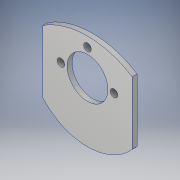
# Autodesk Inventor part: Gear Protection Piece
Saved by Autodesk Inventor 2019.4 (Build 234330000, 330)
## iProperties
Created: 2019-11-02
Part Number: Gear Protection Piece
Material: Aluminum 6061
Document SubType Name: Modeling
Designer: admin
Density: 2.7 g/cm^3
Appearance: Aluminum - Flat
Author: admin
Autodesk Inventor part; units mm, degrees
ref_plane "YZ Plane" through (0, 0, 0) normal (1, 0, 0) x (0, 1, 0)
ref_plane "XZ Plane" through (0, 0, 0) normal (0, 1, 0) x (-1, 0, 0)
ref_plane "XY Plane" through (0, 0, 0) normal (0, 0, 1) x (1, 0, 0)
sketch "Sketch1" plane through (0, 0, 0) normal (0, 0, 1) x (1, 0, 0)
  circle A0 centre (0, 0) radius 12.3
  arc A1 (-26.8669, -23.9619) -> (26.8669, -23.9619) centre (0, 0) ccw
  line L0 (-26.8669, 13.9698) -> (-26.8669, -23.9619)
  line L1 (26.8669, 13.9698) -> (26.8669, -23.9619)
  arc A2 (26.8669, -23.9619) -> (-26.8669, -23.9619) centre (0, 0) ccw construction
  arc A3 (-26.8669, 13.9698) -> (26.8669, 13.9698) centre (0, 0) ccw construction
  arc A4 (26.8669, 13.9698) -> (-26.8669, 13.9698) centre (0, -28.1986) ccw
  line L2 (0, -28.1986) -> (0, 0) construction
  dimension "d0" = 24.6
  dimension "d1" = 72
  dimension "d13" = 50
  constraints: 8 point on circle, 6 end point, 5 centre point, 3 coincident, 2 vertical, 1 parallel
  measures "d0" diameter of A0
  measures "d1" diameter of A1
  measures "d13" radius of A4
extrude "Extrusion1" add sketch "Sketch1" along normal blind 3
sketch "Sketch2" plane through (0, 0, 3) normal (0, 0, 1) x (1, 0, 0)
  circle A0 centre (-16, 0) radius 2.25
  circle A1 centre (16, 0) radius 2.25
  circle A2 centre (0, 16) radius 2.25
  line L0 (0, 0) -> (0, 16) construction
  line L1 (0, 0) -> (16, 0) construction
  line L2 (0, 0) -> (-16, 0) construction
  dimension "d5" = 4.5
  dimension "d6" = 4.5
  dimension "d7" = 4.5
  dimension "d8" = 16
  dimension "d9" = 16
  dimension "d10" = 16
  constraints: 6 end point, 3 centre point, 2 horizontal, 1 coincident, 1 vertical
  measures "d5" diameter of A0
  measures "d6" diameter of A1
  measures "d7" diameter of A2
  measures "d8" distance of L0.start L2.end
  measures "d9" distance of L0.start L1.end
  measures "d10" distance of L0.start L0.end
extrude "Extrusion2" cut sketch "Sketch2" against normal blind 3
equation "\"d9\" = d8"
equation "\"d10\" = d8"
body "Solid1"
